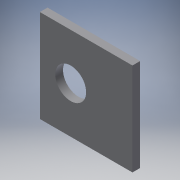
# Autodesk Inventor part: soporte
Saved by Autodesk Inventor 2018 (Build 220112000, 112)
## iProperties
Created: 2021-07-10
Part Number: soporte
Material: Genérico
Document SubType Name: Modeling
Designer: GABRIEL
Density: 1 g/cm^3
Appearance: Valor por defecto
Author: GABRIEL
Autodesk Inventor part; units mm, degrees
ref_plane "YZ Plane" through (0, 0, 0) normal (1, 0, 0) x (0, 1, 0)
ref_plane "XZ Plane" through (0, 0, 0) normal (0, 1, 0) x (-1, 0, 0)
ref_plane "XY Plane" through (0, 0, 0) normal (0, 0, 1) x (1, 0, 0)
sketch "Boceto1" plane through (0, 0, 0) normal (0, 1, 0) x (-1, 0, 0)
  line L0 (0, 0) -> (-80, 0)
  line L1 (-80, 0) -> (-80, -60)
  line L2 (-80, -60) -> (0, -60)
  line L3 (0, -60) -> (0, 0)
  circle A0 centre (-20, -30) radius 10
  dimension "d0" = 80
  dimension "d1" = 60
  dimension "d2" = 20
  dimension "d3" = 30
  dimension "d4" = 20
  constraints: 8 end point, 2 parallel, 1 centre point, 1 horizontal, 1 perpendicular
  measures "d0" distance of L2.end L1.end
  measures "d1" distance of L2.end L0.start
  measures "d2" diameter of A0
  measures "d3" distance from line of L0 A0.centre
  measures "d4" distance from line of L3 A0.centre
extrude "Extrusión1" add sketch "Boceto1" along normal blind 5
